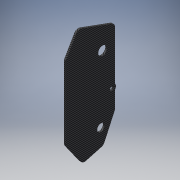
# Autodesk Inventor part: Module Plate 1
Saved by Autodesk Inventor 2019.4 (Build 234330000, 330)
## iProperties
Created: 2019-10-19
Part Number: Module Plate 1
Material: CFRP
Document SubType Name: Modeling
Designer: admin
Density: 1.43 g/cm^3
Appearance: Carbon Fiber
Author: admin
Autodesk Inventor part; units mm, degrees
ref_plane "YZ Plane" through (0, 0, 0) normal (1, 0, 0) x (0, 1, 0)
ref_plane "XZ Plane" through (0, 0, 0) normal (0, 1, 0) x (-1, 0, 0)
ref_plane "XY Plane" through (0, 0, 0) normal (0, 0, 1) x (1, 0, 0)
sketch "Sketch1" plane through (0, 0, 0) normal (1, 0, 0) x (0, 1, 0)
  circle A0 centre (0, 0) radius 76.2 construction
  circle A1 centre (-143.2016, 3.8) radius 50 construction
  line L0 (-143.2016, 3.8) -> (0, 0) construction
  line L1 (-166.1614, -46.2) -> (-106.8647, -46.2) construction
  line L2 (-16.0459, -76.2) -> (40.9165, -76.2) construction
  line L3 (-178.8061, -1.8847) -> (-124.2601, -26.8793)
  line L4 (-124.2601, -26.8793) -> (-86.917, -26.8793)
  line L5 (38.1047, -26.8793) -> (67.356, 53.488)
  line L6 (67.356, 53.488) -> (21.4359, 80)
  line L7 (21.4359, 80) -> (-139.5279, 80)
  line L8 (-139.5279, 80) -> (-191.2312, 43.2818)
  line L9 (-191.2312, 43.2818) -> (-178.8061, -1.8847)
  circle A2 centre (0, 0) radius 9.8
  circle A3 centre (-143.2016, 3.8) radius 8.3
  line L10 (-151.5331, -14.382) -> (-143.2016, 3.8) construction
  arc A4 (-86.917, -26.8793) -> (-75.6033, -26.8793) centre (-81.2601, -19.8793) ccw
  arc A5 (-75.6033, -26.8793) -> (-86.917, -26.8793) centre (-81.2601, -19.8793) ccw construction
  line L11 (-84.6084, -26.8793) -> (-83.9118, -26.8793) construction
  line L12 (-83.9118, -26.8793) -> (-75.6033, -26.8793) construction
  line L13 (-86.917, -26.8793) -> (-84.6084, -26.8793) construction
  line L14 (-75.6033, -26.8793) -> (38.1047, -26.8793)
  circle A6 centre (-81.2601, -19.8793) radius 4
  dimension "d0" = 152.4
  dimension "d1" = 100
  dimension "d2" = 143.252
  dimension "d3" = 30
  dimension "d4" = 20
  dimension "d5" = 19.6
  dimension "d6" = 16.6
  dimension "d7" = 23.099
  dimension "d8" = 60
  dimension "d9" = 130
  dimension "d10" = 110
  dimension "d12" = 155.381
  dimension "d13" = 80
  dimension "d14" = 100
  dimension "d15" = 150
  dimension "d16" = 80
  dimension "d17" = 45
  dimension "d18" = 60
  dimension "d19" = 18
  dimension "d26" = 8
  dimension "d27" = 7
  dimension "d28" = 43
  constraints: 30 end point, 7 centre point, 5 parallel, 4 coincident, 4 point on circle, 2 horizontal, 2 point on line, 2 tangent, 1 midpoint, 1 perpendicular
  measures "d0" diameter of A0
  measures "d1" diameter of A1
  measures "d2" distance of L0.start L0.end
  measures "d3" distance between parallel lines of L2 L1
  measures "d4" distance from line of L0.start L3
  measures "d5" diameter of A2
  measures "d6" diameter of A3
  measures "d7" angle of L0 L3
  measures "d8" distance of L3.start L3.end
  measures "d9" angle of L3 L9
  measures "d10" angle of L9 L8
  measures "d12" angle of L4 L3
  measures "d13" distance from line of A2.centre L7
  measures "d14" angle of L5 L6
  measures "d15" angle of L7 L6
  measures "d16" distance from line of point (0, 0) L6
  measures "d17" distance from line of A2.centre L5
  measures "d18" distance from line of L10.end L8
  measures "d19" diameter of A4
  measures "d26" diameter of A6
  measures "d27" distance from line of L4 A6.centre
  measures "d28" horizontal distance of L3.end A6.centre
extrude "Extrusion1" add sketch "Sketch1" along normal blind 4
fillet "Fillet1" radius 2 2 edges at (2, -86.917, -26.8793) (2, -75.6033, -26.8793)
fillet "Fillet2" radius 10 7 edges at (2, -191.2312, 43.2818) (2, -139.5279, 80) (2, -178.8061, -1.8847) (2, 21.4359, 80) (2, 67.356, 53.488) (2, 38.1047, -26.8793) (2, -124.2601, -26.8793)
body "Solid1"
